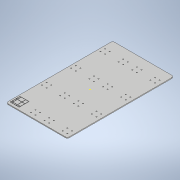
# Autodesk Inventor part: Plastic Inlay
Saved by Autodesk Inventor 2022 (Build 260153000, 153)
## iProperties
Created: 2021-04-06
Part Number: Plastic Inlay
Material: Generic
Document SubType Name: Modeling
Designer: caleb
Density: 1 g/cm^3
Appearance: Default
Author: caleb
Autodesk Inventor part; units mm, degrees
ref_plane "YZ Plane" through (0, 0, 0) normal (1, 0, 0) x (0, 1, 0)
ref_plane "XZ Plane" through (0, 0, 0) normal (0, 1, 0) x (-1, 0, 0)
ref_plane "XY Plane" through (0, 0, 0) normal (0, 0, 1) x (1, 0, 0)
sketch "Sketch1" plane through (0, 0, 0) normal (0, 1, 0) x (-1, 0, 0)
  line L0 (-60, 104.45) -> (60, 104.45)
  line L1 (60, 104.45) -> (60, -104.45)
  line L2 (60, -104.45) -> (-60, -104.45)
  line L3 (-60, -104.45) -> (-60, 104.45)
  line L4 (-60, 104.45) -> (60, -104.45) construction
  line L5 (60, 104.45) -> (-60, -104.45) construction
  point P0 (0, 0)
  dimension "d0" = 120
  dimension "d1" = 208.9
  constraints: 12 end point, 2 midpoint, 2 parallel, 1 horizontal, 1 perpendicular
  measures "d0" distance of L1.end L2.end
  measures "d1" distance of L0.end L1.end
extrude "Extrusion1" add sketch "Sketch1" along normal blind 1.5875
fillet "Fillet1" radius 4 4 edges at (-60, 0.7937, 104.45) (-60, 0.7937, -104.45) (60, 0.7937, -104.45) (60, 0.7937, 104.45)
sketch "Sketch3" plane through (0, 1.5875, 0) normal (0, 1, 0) x (1, 0, 0)
  circle A0 centre (-54.5, -96.95) radius 1
  circle A1 centre (-54.5, -87.95) radius 1
  circle A2 centre (-45.5, -96.95) radius 1
  circle A3 centre (-45.5, -87.95) radius 1
  line L0 (-60, 100.45) -> (-60, -100.45) projected
  line L1 (-56, -104.45) -> (56, -104.45) projected
  circle A4 centre (-54.5, -39.633) radius 1
  circle A5 centre (-54.5, -30.633) radius 1
  circle A6 centre (-45.5, -39.633) radius 1
  circle A7 centre (-45.5, -30.633) radius 1
  circle A8 centre (-54.5, 17.684) radius 1
  circle A9 centre (-54.5, 26.684) radius 1
  circle A10 centre (-45.5, 17.684) radius 1
  circle A11 centre (-45.5, 26.684) radius 1
  circle A12 centre (-54.5, 75.001) radius 1
  circle A13 centre (-54.5, 84.001) radius 1
  circle A14 centre (-45.5, 75.001) radius 1
  circle A15 centre (-45.5, 84.001) radius 1
  circle A16 centre (-18.934, -96.95) radius 1
  circle A17 centre (-18.934, -87.95) radius 1
  circle A18 centre (-9.934, -96.95) radius 1
  circle A19 centre (-9.934, -87.95) radius 1
  circle A20 centre (-18.934, -39.633) radius 1
  circle A21 centre (-18.934, -30.633) radius 1
  circle A22 centre (-9.934, -39.633) radius 1
  circle A23 centre (-9.934, -30.633) radius 1
  circle A24 centre (-18.934, 17.684) radius 1
  circle A25 centre (-18.934, 26.684) radius 1
  circle A26 centre (-9.934, 17.684) radius 1
  circle A27 centre (-9.934, 26.684) radius 1
  circle A28 centre (-18.934, 75.001) radius 1
  circle A29 centre (-18.934, 84.001) radius 1
  circle A30 centre (-9.934, 75.001) radius 1
  circle A31 centre (-9.934, 84.001) radius 1
  circle A32 centre (52.5, -96.95) radius 1
  circle A33 centre (52.5, -87.95) radius 1
  circle A34 centre (43.5, -87.95) radius 1
  circle A35 centre (43.5, -96.95) radius 1
  line L2 (60, -100.45) -> (60, 100.45) projected
  circle A36 centre (43.5, -39.633) radius 1
  circle A37 centre (43.5, -30.633) radius 1
  circle A38 centre (52.5, -39.633) radius 1
  circle A39 centre (52.5, -30.633) radius 1
  circle A40 centre (43.5, 17.684) radius 1
  circle A41 centre (43.5, 26.684) radius 1
  circle A42 centre (52.5, 17.684) radius 1
  circle A43 centre (52.5, 26.684) radius 1
  circle A44 centre (43.5, 75.001) radius 1
  circle A45 centre (43.5, 84.001) radius 1
  circle A46 centre (52.5, 75.001) radius 1
  circle A47 centre (52.5, 84.001) radius 1
  circle A48 centre (7.934, -96.95) radius 1
  circle A49 centre (7.934, -87.95) radius 1
  circle A50 centre (16.934, -96.95) radius 1
  circle A51 centre (16.934, -87.95) radius 1
  circle A52 centre (7.934, -39.633) radius 1
  circle A53 centre (7.934, -30.633) radius 1
  circle A54 centre (16.934, -39.633) radius 1
  circle A55 centre (16.934, -30.633) radius 1
  circle A56 centre (7.934, 17.684) radius 1
  circle A57 centre (7.934, 26.684) radius 1
  circle A58 centre (16.934, 17.684) radius 1
  circle A59 centre (16.934, 26.684) radius 1
  circle A60 centre (7.934, 75.001) radius 1
  circle A61 centre (7.934, 84.001) radius 1
  circle A62 centre (16.934, 75.001) radius 1
  circle A63 centre (16.934, 84.001) radius 1
  point P0 (0, 0)
  dimension "d31" = 2
  dimension "d32" = 9
  dimension "d33" = 9
  dimension "d34" = 5.5
  dimension "d35" = 7.5
  dimension "d38" = 57.317
  dimension "d41" = 35.566
  dimension "d44" = 2
  dimension "d45" = 9
  dimension "d46" = 9
  dimension "d47" = 7.5
  dimension "d48" = 7.5
  dimension "d51" = 57.317
  dimension "d54" = 35.566
  constraints: 64 centre point, 6 equal radius, 4 horizontal alignment, 4 vertical alignment, 2 horizontal, 2 vertical, 112 other
  measures "d31" diameter of A0
  measures "d32" distance of A1.centre A0.centre
  measures "d33" distance of A2.centre A0.centre
  measures "d34" distance from line of L0 A0.centre
  measures "d35" distance from line of L1 A0.centre
  measures "d38" distance of A0.centre A4.centre
  measures "d41" distance of A0.centre A16.centre
  measures "d44" diameter of A32
  measures "d45" distance of A35.centre A32.centre
  measures "d46" distance of A33.centre A32.centre
  measures "d47" distance from line of L2 A33.centre
  measures "d48" distance from line of L1 A32.centre
  measures "d51" distance of A35.centre A36.centre
  measures "d54" distance of A35.centre A48.centre
extrude "Extrusion2" cut sketch "Sketch3" against normal through all
sketch "Sketch4" plane through (0, 1.5875, 0) normal (0, 1, 0) x (1, 0, 0)
  point P0 (0, 0)
sketch "Sketch5" plane through (0, 1.5875, 0) normal (0, 1, 0) x (1, 0, 0)
  line L0 (-57.125, -99.575) -> (-39.375, -99.575)
  line L1 (-39.375, -99.575) -> (-39.375, -80.025)
  line L2 (-39.375, -80.025) -> (-57.125, -80.025)
  line L3 (-57.125, -80.025) -> (-57.125, -99.575)
  circle A0 centre (-54.5, -96.95) radius 1 projected
  circle A1 centre (-54.5, -87.95) radius 1 projected
  line L4 (-39.875, -80.525) -> (-56.625, -80.525)
  line L5 (-56.625, -80.525) -> (-56.625, -99.075)
  line L6 (-56.625, -99.075) -> (-39.875, -99.075)
  line L7 (-39.875, -99.075) -> (-39.875, -80.525)
  line L8 (-56.625, -97.2) -> (-39.875, -97.2)
  line L9 (-39.875, -97.2) -> (-39.875, -96.7)
  line L10 (-39.875, -96.7) -> (-56.625, -96.7)
  line L11 (-56.625, -96.7) -> (-56.625, -97.2)
  line L12 (-56.625, -88.2) -> (-39.875, -88.2)
  line L13 (-39.875, -88.2) -> (-39.875, -87.7)
  line L14 (-39.875, -87.7) -> (-56.625, -87.7)
  line L15 (-56.625, -87.7) -> (-56.625, -88.2)
  line L16 (-54.25, -80.525) -> (-54.75, -80.525)
  line L17 (-54.75, -80.525) -> (-54.75, -99.075)
  line L18 (-54.75, -99.075) -> (-54.25, -99.075)
  line L19 (-54.25, -99.075) -> (-54.25, -80.525)
  line L20 (-45.25, -80.525) -> (-45.75, -80.525)
  line L21 (-45.75, -80.525) -> (-45.75, -99.075)
  line L22 (-45.75, -99.075) -> (-45.25, -99.075)
  line L23 (-45.25, -99.075) -> (-45.25, -80.525)
  circle A2 centre (-45.5, -96.95) radius 1 projected
  point P0 (0, 0)
  point P1 (-54.25, -96.7)
  point P2 (-54.25, -88.2)
  point P3 (-45.75, -88.2)
  point P4 (-45.75, -96.7)
  point P5 (-54.25, -97.2)
  point P6 (-45.75, -97.2)
  point P7 (-45.25, -97.2)
  point P8 (-45.25, -96.7)
  point P9 (-45.25, -88.2)
  point P10 (-45.25, -87.7)
  point P11 (-45.75, -87.7)
  point P12 (-54.25, -87.7)
  point P13 (-54.75, -87.7)
  point P14 (-54.75, -88.2)
  point P15 (-54.75, -96.7)
  point P16 (-54.75, -97.2)
  dimension "d59" = 17.75
  dimension "d60" = 19.55
  dimension "d61" = 2.625
  dimension "d62" = 7.925
  dimension "d63" = 2.625
  dimension "d64" = 0.5
  dimension "d65" = 0.5
  dimension "d66" = 0.5
  dimension "d67" = 0.5
  dimension "d70" = 0.5
  dimension "d71" = 0.5
  dimension "d72" = 0.5
  dimension "d73" = 0.5
  dimension "d74" = 0.25
  dimension "d75" = 0.25
  dimension "d76" = 0.25
  dimension "d77" = 0.25
  constraints: 48 end point, 12 parallel, 8 point on line, 6 horizontal, 6 perpendicular
  measures "d59" distance of L2.end L1.end
  measures "d60" distance of L0.end L1.end
  measures "d61" distance from line of L0 A0.centre
  measures "d62" distance from line of L2 A1.centre
  measures "d63" distance from line of L3 A0.centre
  measures "d64" distance between parallel lines of L3 L5
  measures "d65" distance between parallel lines of L2 L4
  measures "d66" distance between parallel lines of L1 L7
  measures "d67" distance between parallel lines of L0 L6
  measures "d70" distance between parallel lines of L17 L19
  measures "d71" distance between parallel lines of L12 L14
  measures "d72" distance between parallel lines of L8 L10
  measures "d73" distance between parallel lines of L23 L21
  measures "d74" distance from line of L8 A0.centre
  measures "d75" distance from line of L17 A0.centre
  measures "d76" distance from line of L12 A1.centre
  measures "d77" distance from line of L21 A2.centre
extrude "Extrusion3" cut sketch "Sketch5" against normal blind 1 contours L3 L2 L1 L0 | A0 L8 L19 L10 | A0 L10 A2 L8 | L19 L10 L17 A0 | A0 L17 A1 L19 | L10 L21 L8 A2 | L19 L8 L17 L10 | L19 L6 L17 A0 | A0 L17 L8 L19 | A1 L17 L12 L19 | L21 A2 L23 L10 | L10 L23 L8 L21 | L21 L12 L23 A2 | L17 L8 A0 L10 | L8 L23 A2 L21 | A2 L23 L6 L21 | A0 L8 L5 L10 | L12 L19 L14 A1 | A1 L14 L21 L12 | L12 L17 L14 L19 | L10 A2 L8 L23 | L21 L14 L23 L12 | L12 L5 L14 A1 | A1 L14 L17 L12 | L14 L17 A1 L19 | L10 L7 L8 A2 | L23 L14 L7 L12 | L21 L4 L23 L14 | A1 L17 L4 L19
equation "\"d44\" = d31"
equation "\"d45\" = d33"
equation "\"d46\" = d32"
equation "\"d48\" = d35"
equation "\"d51\" = d38"
equation "\"d54\" = d41"
equation "\"d63\" = d61"
equation "\"d65\" = d64"
equation "\"d66\" = d64"
equation "\"d67\" = d64"
equation "\"d70\" = d64"
equation "\"d71\" = d64"
equation "\"d72\" = d64"
equation "\"d73\" = d64"
body "Solid1"
